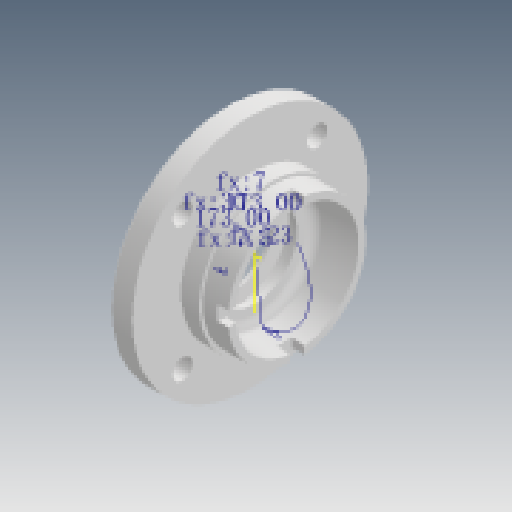
# Autodesk Inventor part: 低速轴承透盖
Saved by Autodesk Inventor 2025 (Build 290162000, 162)
## iProperties
Created: 2025-03-14
Part Number: 低速轴承透盖
Material: 常规
Document SubType Name: Modeling
Designer: ASUS
Density: 1 g/cm^3
Appearance: 默认
Author: ASUS
Autodesk Inventor part; units mm, degrees
ref_plane "YZ Plane" through (0, 0, 0) normal (1, 0, 0) x (0, 1, 0)
ref_plane "XZ Plane" through (0, 0, 0) normal (0, 1, 0) x (-1, 0, 0)
ref_plane "XY Plane" through (0, 0, 0) normal (0, 0, 1) x (1, 0, 0)
sketch "草图1" plane through (0, 0, 0) normal (0, 1, 0) x (-1, 0, 0)
  line L0 (0, 65) -> (-12, 65)
  line L1 (-12, 65) -> (-12, 38)
  line L2 (-12, 38) -> (-14.5, 38)
  line L3 (-14.5, 38) -> (-14.5, 40)
  line L4 (-14.5, 40) -> (-24, 40)
  line L5 (-24, 40) -> (-24, 38)
  line L6 (-24, 38) -> (-38, 38)
  line L7 (-38, 38) -> (-38, 0)
  line L8 (-38, 0) -> (0, 0)
  line L9 (0, 0) -> (0, 65)
  line L10 (0, 38) -> (-1, 37)
  line L11 (-1, 37) -> (-1, 0)
  line L12 (-38, 34) -> (-15, 31.6998)
  line L13 (-15, 31.6998) -> (-15, 0)
  line L14 (7.6, 0) -> (-45.6, 0) projected
  dimension "d2" = 65
  dimension "d4" = 26
  dimension "d5" = 12
  dimension "d6" = 40
  dimension "d7" = 38
  dimension "d8" = 12
  dimension "d9" = 2.5
  dimension "d10" = 38
  dimension "d11" = 45
  dimension "d12" = 1
  dimension "d13" = 15
  dimension "d14" = 34
  dimension "d15" = 84.289
  constraints: 28 end point, 10 perpendicular, 6 point on line, 1 horizontal
  measures "d2" distance of L8.end L0.start
  measures "d4" distance between parallel lines of L7 L1
  measures "d5" distance of L0.start L0.end
  measures "d6" distance between parallel lines of L8 L4
  measures "d7" distance between parallel lines of L8 L6
  measures "d8" distance between parallel lines of L5 L1
  measures "d9" distance of L1.end L2.end
  measures "d10" distance from line of L8 L10.start
  measures "d11" angle of L9 L10
  measures "d12" distance between parallel lines of L9 L11
  measures "d13" distance between parallel lines of L9 L13
  measures "d14" distance from line of L8 L12.start
  measures "d15" angle of L7 L12
revolve "旋转1" add sketch "草图1" angle 360 about axis through (-10, 0, 0) along (1, 0, 0) contours L9 L10 L11 L8 L13 L12 L7 L6 L5 L4 L3 L2 L1 L0
sketch "草图2" plane through (0, 0, 0) normal (0, 1, 0) x (-1, 0, 0)
  line L0 (-24, 38) -> (-38, 38) projected
  line L1 (-39, 38) -> (-32, 38)
  line L2 (-32, 38) -> (-32, -20)
  line L3 (-32, -20) -> (-39, -20)
  line L4 (-39, -20) -> (-39, 38)
  point P0 (0, 0)
  dimension "d17" = 7
  constraints: 8 end point, 2 parallel, 1 horizontal, 1 perpendicular, 1 point on line
  measures "d17" distance between parallel lines of L2 L4
extrude "拉伸1" cut sketch "草图2" along normal mid plane 8
sketch "草图3" plane through (0, 0, 0) normal (0, 0, 1) x (1, 0, 0)
  line L0 (38, 4) -> (38, 38) projected
  line L1 (24, -38) -> (38, -38) projected
  line L2 (38, 38) -> (31, 38)
  line L3 (31, 38) -> (31, -38)
  line L4 (31, -38) -> (38, -38)
  line L5 (38, -38) -> (38, 38)
  point P0 (0, 0)
  point P1 (38, -4)
  dimension "d20" = 7
  constraints: 8 end point, 2 parallel, 1 horizontal, 1 midpoint, 1 perpendicular
  measures "d20" distance between parallel lines of L5 L3
extrude "拉伸2" cut sketch "草图3" along normal mid plane 8
sketch "草图4" plane through (0, 0, 0) normal (-1, 0, 0) x (0, 0, 1)
  circle A0 centre (37.1231, 37.1231) radius 5.5
  circle A1 centre (-37.1231, 37.1231) radius 5.5
  circle A2 centre (-37.1231, -37.1231) radius 5.5
  circle A3 centre (37.1231, -37.1231) radius 5.5
  line L0 (37.1231, 37.1231) -> (0, 0)
  line L1 (0, -91) -> (0, 91) projected
  dimension "d23" = 11
  dimension "d24" = 52.5
  dimension "d27" = 360
  dimension "d42" = 45
  constraints: 4 centre point, 2 end point, 9 other
  measures "d23" diameter of A0
  measures "d24" distance of L0.end L0.start
  measures "d42" angle of L1 L0
extrude "拉伸3" cut sketch "草图4" against normal up to surface (12 mm away)
chamfer "倒角1" distance 1 angle 45 1 edges at (0, 0, -65)
fillet "圆角1" radius 5 1 edges at (15, 0, -31.6998)
sketch "草图5" plane through (0, 0, 0) normal (0, 0, 1) x (1, 0, 0)
  line L0 (0, -38) -> (0, 38) projected
  line L1 (0, 23) -> (3.1405, 23)
  line L2 (3.1405, 23) -> (4, 30)
  line L3 (4, 30) -> (11, 30)
  line L4 (11, 30) -> (11.8595, 23)
  line L5 (11.8595, 23) -> (15, 23)
  line L6 (15, 27.1749) -> (15, -27.1749) projected
  line L7 (0, 23) -> (0, 0)
  line L8 (0, 0) -> (15, 0)
  line L9 (15, 23) -> (15, 0)
  line L10 (-3, 0) -> (18, 0) projected
  point P0 (7.5, 30)
  dimension "d35" = 23
  dimension "d36" = 30
  dimension "d37" = 7
  dimension "d38" = 7
  dimension "d39" = 7
  dimension "d40" = 7.5
  constraints: 16 end point, 4 point on line, 2 midpoint, 2 perpendicular, 1 horizontal, 1 parallel
  measures "d35" distance between parallel lines of L8 L5
  measures "d36" distance between parallel lines of L8 L3
  measures "d37" distance of L2.end L3.end
  measures "d38" angle of L0 L2
  measures "d39" angle of L6 L4
  measures "d40" distance from line of L0 point (7.5, 30)
revolve "旋转2" cut sketch "草图5" angle 360 about axis through (-10, 0, 0) along (1, 0, 0)
equation "\"d2\" = 0.5 * D2"
equation "\"d4\" = M"
equation "\"d5\" = e"
equation "\"d6\" = 0.5 * D"
equation "\"d7\" = 0.5 * D_d"
equation "\"d8\" = e1"
equation "\"d10\" = 0.5 * D_d"
equation "\"d13\" = b1"
equation "\"d14\" = 0.5 * D4"
equation "\"d17\" = h_b"
equation "\"d18\" = b"
equation "\"d20\" = h_b"
equation "\"d21\" = b"
equation "\"d23\" = d0"
equation "\"d24\" = 0.5 * D0"
equation "\"d29\" = b"
equation "\"d35\" = 0.5 * d1"
equation "\"d36\" = 0.5 * d1_D0"
equation "\"d37\" = d1_b"
equation "\"d40\" = 0.5 * b1"
equation "\"d0\" = 11"
equation "\"D0\" = 105"
equation "\"D4\" = 68"
equation "\"D_d\" = 76"
equation "\"e\" = 12"
equation "\"e1\" = 12"
equation "\"b\" = 8"
equation "\"h_b\" = 7"
equation "\"M\" = 26"
equation "\"b1\" = 15"
equation "\"d1\" = 46"
equation "\"d1_b\" = 7"
equation "\"D2\" = 130"
equation "\"D\" = 80"
equation "\"d1_D0\" = 60"
